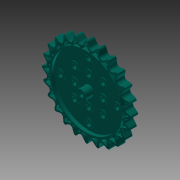
# Autodesk Inventor part: 276-2252
Saved by Autodesk Inventor 2013 (Build 170138000, 138)
## iProperties
Category: Motion
Company: Autodesk Inc.
Created: 2012-03-01
Part Number: 276-2252
Document SubType Name: Modeling
Designer: Autodesk Inc.
Density: 1.42 g/cm^3
Material: Acetal Resin, White
Catalog Web Link: http://www.vexrobotics.com/276-2252.html
Vendor: VEX
Mass: 20.1028 g
Surface Area: 159.433 cm^2
Volume: 14.1569 cm^3
Author: Autodesk Inc.
Autodesk Inventor part; units mm, degrees
ref_plane "YZ Plane" through (0, 0, 0) normal (1, 0, 0) x (0, 1, 0)
ref_plane "XZ Plane" through (0, 0, 0) normal (0, 1, 0) x (-1, 0, 0)
ref_plane "XY Plane" through (0, 0, 0) normal (0, 0, 1) x (1, 0, 0)
sketch "Sketch1" plane through (0, 0, 0) normal (0, 0, 1) x (1, 0, 0)
  circle A0 centre (0, -25.4) radius 2.2225
  circle A1 centre (-12.7, -12.7) radius 2.2225
  circle A2 centre (0, -12.7) radius 2.2225
  circle A3 centre (12.7, -12.7) radius 2.2225
  circle A4 centre (25.4, 0) radius 2.2225
  circle A5 centre (-25.4, 0) radius 2.2225
  circle A6 centre (12.7, 0) radius 2.2225
  circle A7 centre (12.7, 12.7) radius 2.2225
  circle A8 centre (0, 25.4) radius 2.2225
  circle A9 centre (-12.7, 12.7) radius 2.2225
  circle A10 centre (-12.7, 0) radius 2.2225
  circle A11 centre (0, 12.7) radius 2.2225
  line L0 (-1.5875, 1.5875) -> (-1.5875, -1.5875)
  line L1 (-1.5875, -1.5875) -> (1.5875, -1.5875)
  line L2 (1.5875, -1.5875) -> (1.5875, 1.5875)
  line L3 (1.5875, 1.5875) -> (-1.5875, 1.5875)
  arc A12 (35.6037, 6.8783) -> (36.1708, 2.571) centre (37.2166, 4.8997) ccw
  line L4 (36.1708, 2.571) -> (38.9403, 1.3272)
  arc A13 (40.0602, 0.0966) -> (38.9403, 1.3272) centre (38.0859, -0.5752) ccw
  arc A14 (40.0602, -0.0966) -> (40.0602, 0.0966) centre (39.7762, 0) ccw
  arc A15 (38.9403, -1.3272) -> (40.0602, -0.0966) centre (38.0859, 0.5752) ccw
  line L5 (38.9403, -1.3272) -> (36.1708, -2.571)
  arc A16 (36.1708, -2.571) -> (35.6037, -6.8783) centre (37.2166, -4.8997) ccw
  line L6 (35.6037, -6.8783) -> (37.9569, -8.7965)
  arc A17 (38.7202, -10.275) -> (37.9569, -8.7965) centre (36.6392, -10.413) ccw
  arc A18 (38.6701, -10.4617) -> (38.7202, -10.275) centre (38.4208, -10.2948) ccw
  arc A19 (37.2699, -11.3605) -> (38.6701, -10.4617) centre (36.937, -9.3017) ccw
  line L7 (37.2699, -11.3605) -> (34.2729, -11.8451)
  arc A20 (34.2729, -11.8451) -> (32.6103, -15.8588) centre (34.6804, -14.3651) ccw
  line L8 (32.6103, -15.8588) -> (34.3869, -18.3207)
  arc A21 (34.7414, -19.9464) -> (34.3869, -18.3207) centre (32.6957, -19.5411) ccw
  arc A22 (34.6448, -20.1138) -> (34.7414, -19.9464) centre (34.4472, -19.8881) ccw
  arc A23 (33.0597, -20.6195) -> (34.6448, -20.1138) centre (33.2709, -18.5448) ccw
  line L9 (33.0597, -20.6195) -> (30.0393, -20.312)
  arc A24 (30.0393, -20.312) -> (27.3946, -23.7586) centre (29.7807, -22.8515) ccw
  line L10 (27.3946, -23.7586) -> (28.4734, -26.5964)
  arc A25 (28.3952, -28.2585) -> (28.4734, -26.5964) centre (26.524, -27.3375) ccw
  arc A26 (28.2585, -28.3952) -> (28.3952, -28.2585) centre (28.126, -28.126) ccw
  arc A27 (26.5964, -28.4734) -> (28.2585, -28.3952) centre (27.3375, -26.524) ccw
  line L11 (26.5964, -28.4734) -> (23.7586, -27.3946)
  arc A28 (23.7586, -27.3946) -> (20.312, -30.0393) centre (22.8515, -29.7807) ccw
  line L12 (20.312, -30.0393) -> (20.6195, -33.0597)
  arc A29 (20.1138, -34.6448) -> (20.6195, -33.0597) centre (18.5448, -33.2709) ccw
  arc A30 (19.9464, -34.7414) -> (20.1138, -34.6448) centre (19.8881, -34.4472) ccw
  arc A31 (18.3207, -34.3869) -> (19.9464, -34.7414) centre (19.5411, -32.6957) ccw
  line L13 (18.3207, -34.3869) -> (15.8588, -32.6103)
  arc A32 (15.8588, -32.6103) -> (11.8451, -34.2729) centre (14.3651, -34.6804) ccw
  line L14 (11.8451, -34.2729) -> (11.3605, -37.2699)
  arc A33 (10.4617, -38.6701) -> (11.3605, -37.2699) centre (9.3017, -36.937) ccw
  arc A34 (10.275, -38.7202) -> (10.4617, -38.6701) centre (10.2948, -38.4208) ccw
  arc A35 (8.7965, -37.9569) -> (10.275, -38.7202) centre (10.413, -36.6392) ccw
  line L15 (8.7965, -37.9569) -> (6.8783, -35.6037)
  arc A36 (6.8783, -35.6037) -> (2.571, -36.1708) centre (4.8997, -37.2166) ccw
  line L16 (2.571, -36.1708) -> (1.3272, -38.9403)
  arc A37 (0.0966, -40.0602) -> (1.3272, -38.9403) centre (-0.5752, -38.0859) ccw
  arc A38 (-0.0966, -40.0602) -> (0.0966, -40.0602) centre (0, -39.7762) ccw
  arc A39 (-1.3272, -38.9403) -> (-0.0966, -40.0602) centre (0.5752, -38.0859) ccw
  line L17 (-1.3272, -38.9403) -> (-2.571, -36.1708)
  arc A40 (-2.571, -36.1708) -> (-6.8783, -35.6037) centre (-4.8997, -37.2166) ccw
  line L18 (-6.8783, -35.6037) -> (-8.7965, -37.9569)
  arc A41 (-10.275, -38.7202) -> (-8.7965, -37.9569) centre (-10.413, -36.6392) ccw
  arc A42 (-10.4617, -38.6701) -> (-10.275, -38.7202) centre (-10.2948, -38.4208) ccw
  arc A43 (-11.3605, -37.2699) -> (-10.4617, -38.6701) centre (-9.3017, -36.937) ccw
  line L19 (-11.3605, -37.2699) -> (-11.8451, -34.2729)
  arc A44 (-11.8451, -34.2729) -> (-15.8588, -32.6103) centre (-14.3651, -34.6804) ccw
  line L20 (-15.8588, -32.6103) -> (-18.3207, -34.3869)
  arc A45 (-19.9464, -34.7414) -> (-18.3207, -34.3869) centre (-19.5411, -32.6957) ccw
  arc A46 (-20.1138, -34.6448) -> (-19.9464, -34.7414) centre (-19.8881, -34.4472) ccw
  arc A47 (-20.6195, -33.0597) -> (-20.1138, -34.6448) centre (-18.5448, -33.2709) ccw
  line L21 (-20.6195, -33.0597) -> (-20.312, -30.0393)
  arc A48 (-20.312, -30.0393) -> (-23.7586, -27.3946) centre (-22.8515, -29.7807) ccw
  line L22 (-23.7586, -27.3946) -> (-26.5964, -28.4734)
  arc A49 (-28.2585, -28.3952) -> (-26.5964, -28.4734) centre (-27.3375, -26.524) ccw
  arc A50 (-28.3952, -28.2585) -> (-28.2585, -28.3952) centre (-28.126, -28.126) ccw
  arc A51 (-28.4734, -26.5964) -> (-28.3952, -28.2585) centre (-26.524, -27.3375) ccw
  line L23 (-28.4734, -26.5964) -> (-27.3946, -23.7586)
  arc A52 (-27.3946, -23.7586) -> (-30.0393, -20.312) centre (-29.7807, -22.8515) ccw
  line L24 (-30.0393, -20.312) -> (-33.0597, -20.6195)
  arc A53 (-34.6448, -20.1138) -> (-33.0597, -20.6195) centre (-33.2709, -18.5448) ccw
  arc A54 (-34.7414, -19.9464) -> (-34.6448, -20.1138) centre (-34.4472, -19.8881) ccw
  arc A55 (-34.3869, -18.3207) -> (-34.7414, -19.9464) centre (-32.6957, -19.5411) ccw
  line L25 (-34.3869, -18.3207) -> (-32.6103, -15.8588)
  arc A56 (-32.6103, -15.8588) -> (-34.2729, -11.8451) centre (-34.6804, -14.3651) ccw
  line L26 (-34.2729, -11.8451) -> (-37.2699, -11.3605)
  arc A57 (-38.6701, -10.4617) -> (-37.2699, -11.3605) centre (-36.937, -9.3017) ccw
  arc A58 (-38.7202, -10.275) -> (-38.6701, -10.4617) centre (-38.4208, -10.2948) ccw
  arc A59 (-37.9569, -8.7965) -> (-38.7202, -10.275) centre (-36.6392, -10.413) ccw
  line L27 (-37.9569, -8.7965) -> (-35.6037, -6.8783)
  arc A60 (-35.6037, -6.8783) -> (-36.1708, -2.571) centre (-37.2166, -4.8997) ccw
  line L28 (-36.1708, -2.571) -> (-38.9403, -1.3272)
  arc A61 (-40.0602, -0.0966) -> (-38.9403, -1.3272) centre (-38.0859, 0.5752) ccw
  arc A62 (-40.0602, 0.0966) -> (-40.0602, -0.0966) centre (-39.7762, 0) ccw
  arc A63 (-38.9403, 1.3272) -> (-40.0602, 0.0966) centre (-38.0859, -0.5752) ccw
  line L29 (-38.9403, 1.3272) -> (-36.1708, 2.571)
  arc A64 (-36.1708, 2.571) -> (-35.6037, 6.8783) centre (-37.2166, 4.8997) ccw
  line L30 (-35.6037, 6.8783) -> (-37.9569, 8.7965)
  arc A65 (-38.7202, 10.275) -> (-37.9569, 8.7965) centre (-36.6392, 10.413) ccw
  arc A66 (-38.6701, 10.4617) -> (-38.7202, 10.275) centre (-38.4208, 10.2948) ccw
  arc A67 (-37.2699, 11.3605) -> (-38.6701, 10.4617) centre (-36.937, 9.3017) ccw
  line L31 (-37.2699, 11.3605) -> (-34.2729, 11.8451)
  arc A68 (-34.2729, 11.8451) -> (-32.6103, 15.8588) centre (-34.6804, 14.3651) ccw
  line L32 (-32.6103, 15.8588) -> (-34.3869, 18.3207)
  arc A69 (-34.7414, 19.9464) -> (-34.3869, 18.3207) centre (-32.6957, 19.5411) ccw
  arc A70 (-34.6448, 20.1138) -> (-34.7414, 19.9464) centre (-34.4472, 19.8881) ccw
  arc A71 (-33.0597, 20.6195) -> (-34.6448, 20.1138) centre (-33.2709, 18.5448) ccw
  line L33 (-33.0597, 20.6195) -> (-30.0393, 20.312)
  arc A72 (-30.0393, 20.312) -> (-27.3946, 23.7586) centre (-29.7807, 22.8515) ccw
  line L34 (-27.3946, 23.7586) -> (-28.4734, 26.5964)
  arc A73 (-28.3952, 28.2585) -> (-28.4734, 26.5964) centre (-26.524, 27.3375) ccw
  arc A74 (-28.2585, 28.3952) -> (-28.3952, 28.2585) centre (-28.126, 28.126) ccw
  arc A75 (-26.5964, 28.4734) -> (-28.2585, 28.3952) centre (-27.3375, 26.524) ccw
  line L35 (-26.5964, 28.4734) -> (-23.7586, 27.3946)
  arc A76 (-23.7586, 27.3946) -> (-20.312, 30.0393) centre (-22.8515, 29.7807) ccw
  line L36 (-20.312, 30.0393) -> (-20.6195, 33.0597)
  arc A77 (-20.1138, 34.6448) -> (-20.6195, 33.0597) centre (-18.5448, 33.2709) ccw
  arc A78 (-19.9464, 34.7414) -> (-20.1138, 34.6448) centre (-19.8881, 34.4472) ccw
  arc A79 (-18.3207, 34.3869) -> (-19.9464, 34.7414) centre (-19.5411, 32.6957) ccw
  line L37 (-18.3207, 34.3869) -> (-15.8588, 32.6103)
  arc A80 (-15.8588, 32.6103) -> (-11.8451, 34.2729) centre (-14.3651, 34.6804) ccw
  line L38 (-11.8451, 34.2729) -> (-11.3605, 37.2699)
  arc A81 (-10.4617, 38.6701) -> (-11.3605, 37.2699) centre (-9.3017, 36.937) ccw
  arc A82 (-10.275, 38.7202) -> (-10.4617, 38.6701) centre (-10.2948, 38.4208) ccw
  arc A83 (-8.7965, 37.9569) -> (-10.275, 38.7202) centre (-10.413, 36.6392) ccw
  line L39 (-8.7965, 37.9569) -> (-6.8783, 35.6037)
  arc A84 (-6.8783, 35.6037) -> (-2.571, 36.1708) centre (-4.8997, 37.2166) ccw
  line L40 (-2.571, 36.1708) -> (-1.3272, 38.9403)
  arc A85 (-0.0966, 40.0602) -> (-1.3272, 38.9403) centre (0.5752, 38.0859) ccw
  arc A86 (0.0966, 40.0602) -> (-0.0966, 40.0602) centre (0, 39.7762) ccw
  arc A87 (1.3272, 38.9403) -> (0.0966, 40.0602) centre (-0.5752, 38.0859) ccw
  line L41 (1.3272, 38.9403) -> (2.571, 36.1708)
  arc A88 (2.571, 36.1708) -> (6.8783, 35.6037) centre (4.8997, 37.2166) ccw
  line L42 (6.8783, 35.6037) -> (8.7965, 37.9569)
  arc A89 (10.275, 38.7202) -> (8.7965, 37.9569) centre (10.413, 36.6392) ccw
  arc A90 (10.4617, 38.6701) -> (10.275, 38.7202) centre (10.2948, 38.4208) ccw
  arc A91 (11.3605, 37.2699) -> (10.4617, 38.6701) centre (9.3017, 36.937) ccw
  line L43 (11.3605, 37.2699) -> (11.8451, 34.2729)
  arc A92 (11.8451, 34.2729) -> (15.8588, 32.6103) centre (14.3651, 34.6804) ccw
  line L44 (15.8588, 32.6103) -> (18.3207, 34.3869)
  arc A93 (19.9464, 34.7414) -> (18.3207, 34.3869) centre (19.5411, 32.6957) ccw
  arc A94 (20.1138, 34.6448) -> (19.9464, 34.7414) centre (19.8881, 34.4472) ccw
  arc A95 (20.6195, 33.0597) -> (20.1138, 34.6448) centre (18.5448, 33.2709) ccw
  line L45 (20.6195, 33.0597) -> (20.312, 30.0393)
  arc A96 (20.312, 30.0393) -> (23.7586, 27.3946) centre (22.8515, 29.7807) ccw
  line L46 (23.7586, 27.3946) -> (26.5964, 28.4734)
  arc A97 (28.2585, 28.3952) -> (26.5964, 28.4734) centre (27.3375, 26.524) ccw
  arc A98 (28.3952, 28.2585) -> (28.2585, 28.3952) centre (28.126, 28.126) ccw
  arc A99 (28.4734, 26.5964) -> (28.3952, 28.2585) centre (26.524, 27.3375) ccw
  line L47 (28.4734, 26.5964) -> (27.3946, 23.7586)
  arc A100 (27.3946, 23.7586) -> (30.0393, 20.312) centre (29.7807, 22.8515) ccw
  line L48 (30.0393, 20.312) -> (33.0597, 20.6195)
  arc A101 (34.6448, 20.1138) -> (33.0597, 20.6195) centre (33.2709, 18.5448) ccw
  arc A102 (34.7414, 19.9464) -> (34.6448, 20.1138) centre (34.4472, 19.8881) ccw
  arc A103 (34.3869, 18.3207) -> (34.7414, 19.9464) centre (32.6957, 19.5411) ccw
  line L49 (34.3869, 18.3207) -> (32.6103, 15.8588)
  arc A104 (32.6103, 15.8588) -> (34.2729, 11.8451) centre (34.6804, 14.3651) ccw
  line L50 (34.2729, 11.8451) -> (37.2699, 11.3605)
  arc A105 (38.6701, 10.4617) -> (37.2699, 11.3605) centre (36.937, 9.3017) ccw
  arc A106 (38.7202, 10.275) -> (38.6701, 10.4617) centre (38.4208, 10.2948) ccw
  arc A107 (37.9569, 8.7965) -> (38.7202, 10.275) centre (36.6392, 10.413) ccw
  line L51 (37.9569, 8.7965) -> (35.6037, 6.8783)
  point P0 (0, 0)
  point P1 (0, 0)
  constraints: 192 point on circle, 108 centre point, 104 end point
extrude "Extrusion1" add sketch "Sketch1" along normal mid plane 7.62 contours A0 | A1 | A2 | A3 | A4 | A5 | A6 | A7 | A8 | A9 | A10 | A11 | L3 L2 L1 L0 | A12 L4 A13 A14 A15 L5 A16 L6 A17 A18 A19 L7 A20 L8 A21 A22 A23 L9 A24 L10 A25 A26 A27 L11 A28 L12 A29 A30 A31 L13 A32 L14 A33 A34 A35 L15 A36 L16 A37 A38 A39 L17 A40 L18 A41 A42 A43 L19 A44 L20 A45 A46 A47 L21 A48 L22 A49 A50 A51 L23 A52 L24 A53 A54 A55 L25 A56 L26 A57 A58 A59 L27 A60 L28 A61 A62 A63 L29 A64 L30 A65 A66 A67 L31 A68 L32 A69 A70 A71 L33 A72 L34 A73 A74 A75 L35 A76 L36 A77 A78 A79 L37 A80 L38 A81 A82 A83 L39 A84 L40 A85 A86 A87 L41 A88 L42 A89 A90 A91 L43 A92 L44 A93 A94 A95 L45 A96 L46 A97 A98 A99 L47 A100 L48 A101 A102 A103 L49 A104 L50 A105 A106 A107 L51
sketch "Sketch2" plane through (0, 0, 3.81) normal (0, 0, 1) x (1, 0, 0)
  circle A0 centre (0, 0) radius 31.0007
  dimension "d2" = 62.0014
  constraints: 1 centre point, 1 coincident
  measures "d2" diameter of A0
extrude "Extrusion2" cut sketch "Sketch2" against normal blind 2.8194
sketch "Sketch3" plane through (0, 0, 0.9906) normal (0, 0, 1) x (1, 0, 0)
  circle A0 centre (0, 0) radius 31.0007 projected
  circle A1 centre (0, 0) radius 4.4958
  dimension "d5" = 8.9916
  constraints: 1 centre point, 1 coincident
  measures "d5" diameter of A1
extrude "Extrusion3" add sketch "Sketch3" along normal blind 6.9342 contours A1
sketch "Sketch4" plane through (0, 0, 0) normal (1, 0, 0) x (0, 1, 0)
  line L0 (40.0602, -3.81) -> (40.0602, 3.81) projected
  line L1 (36.1708, 3.81) -> (38.9403, 3.81) projected
  line L2 (38.9403, 3.81) -> (40.0602, 3.81) projected
  line L3 (34.2729, 3.81) -> (32.1277, 3.81) projected
  line L4 (36.1708, 3.81) -> (34.6639, 3.81) projected
  line L5 (40.0762, -3.81) -> (40.0762, 3.81) projected
  line L6 (40.0762, 3.81) -> (40.0762, 3.0734)
  line L7 (40.0762, 3.0734) -> (35.8852, 3.81)
  line L8 (35.8852, 3.81) -> (40.0762, 3.81)
  line L9 (0, -5.334) -> (0, 5.334) projected
  point P0 (0, 0)
  point P1 (32.6103, 3.81)
  point P2 (35.6037, 3.81)
  dimension "d8" = 0.7366
  dimension "d9" = 4.191
  constraints: 6 end point, 2 point on line, 1 perpendicular
  measures "d8" distance of L6.end L5.end
  measures "d9" distance of L7.end L5.end
revolve "Revolution1" cut sketch "Sketch4" angle 360 about axis through (0, 0, -10) along (0, 0, 1)
sketch "Sketch5" plane through (0, 0, 3.81) normal (0, 0, 1) x (1, 0, 0)
  line L0 (-36.1588, 0.9321) -> (-35.5563, 1.2027)
  arc A0 (-35.5563, 1.2027) -> (-33.3659, 3.6362) centre (-37.2166, 4.8997) ccw
  line L1 (-33.3659, 3.6362) -> (-32.3113, 3.4974)
  arc A1 (-32.3113, 3.4974) -> (-32.3113, -3.4974) centre (0, 0) ccw
  line L2 (-32.3113, -3.4974) -> (-33.3659, -3.6362)
  arc A2 (-33.3659, -3.6362) -> (-35.5563, -1.2027) centre (-37.2166, -4.8997) ccw
  line L3 (-36.1588, -0.9321) -> (-35.5563, -1.2027)
  line L4 (-38.2342, 0) -> (-36.1588, 0.9321)
  ellipse E0 centre (-37.2141, 4.8919) end of major axis (-34.7934, 5.6895) minor radius 2.5445 (-36.1708, 2.571) -> (-36.0761, 2.6159) ccw
  spline S0 degree 3 poles (-38.9403, 1.3272) (-38.6326, 1.4654) (-38.3249, 1.6036) (-38.0172, 1.7418) (-37.7096, 1.8799) (-37.4018, 2.0181) (-37.0941, 2.1564) (-36.7863, 2.2946) (-36.4786, 2.4328) (-36.1708, 2.571) knots 0 0 0 0 0.333333 0.333333 0.333333 0.666667 0.666667 0.666667 1 1 1 1
  spline S1 degree 3 poles (-40.0602, 0.0966) (-40.0458, 0.1387) (-40.0301, 0.1804) (-39.9033, 0.4873) (-39.7357, 0.7287) (-39.3736, 1.082) (-39.1668, 1.2255) (-38.9403, 1.3272) knots 0 0 0 0 0.076332 0.076332 0.569765 0.569765 1 1 1 1
  spline S2 degree 3 poles (-40.0602, 0.0966) (-40.0709, 0.065) (-40.0762, 0.0316) (-40.0762, -0.0316) (-40.0709, -0.065) (-40.0602, -0.0966) knots 0 0 0 0 0.5 0.5 1 1 1 1
  spline S3 degree 3 poles (-38.9403, -1.3272) (-39.1668, -1.2255) (-39.3736, -1.082) (-39.7357, -0.7287) (-39.9033, -0.4873) (-40.0301, -0.1804) (-40.0458, -0.1387) (-40.0602, -0.0966) knots 0 0 0 0 0.430235 0.430235 0.923668 0.923668 1 1 1 1
  spline S4 degree 3 poles (-38.9403, -1.3272) (-38.6245, -1.469) (-38.3114, -1.6097) (-38.001, -1.7491) (-37.6905, -1.8885) (-37.3828, -2.0267) (-37.0778, -2.1637) (-36.7728, -2.3007) (-36.4704, -2.4365) (-36.1708, -2.571) knots 0 0 0 0 0.333333 0.333333 0.333333 0.666667 0.666667 0.666667 1 1 1 1
  ellipse E1 centre (-37.2137, -4.8911) end of major axis (-34.8027, -5.7161) minor radius 2.5436 (-36.0761, -2.6159) -> (-36.1708, -2.571) ccw
  line L5 (-36.1588, -0.9321) -> (-38.2342, 0)
  constraints: 71 coincident, 12 end point, 6 point on circle, 3 centre point, 1 vertical alignment, 20 other
extrude "Extrusion4" cut sketch "Sketch5" against normal blind 2.8194
fillet "Fillet1" radius 0.3048 12 edges at (-38.2342, 0, 2.1939) (-37.1965, -0.466, 0.9906) (-34.2044, -2.1884, 0.9906) (-34.2044, 2.1884, 0.9906) (-35.8575, 1.0674, 0.9906) (-33.3659, 3.6362, 2.4003) (-32.3113, 3.4974, 2.4003) (-32.3113, -3.4974, 2.4003) (-32.8386, 3.5668, 0.9906) (-32.8386, -3.5668, 0.9906) (-33.3659, -3.6362, 2.4003) (-32.5, 0, 0.9906)
pattern_circular "Circular Pattern1" count 24 over 360 about axis through (0, 0, 0.9906) along (0, 0, 1) of "Extrusion4", "Fillet1"
fillet "Fillet2" radius 0.3048 3 edges at (-31.0007, 0, 0.9906) (-4.4958, 0, 0.9906) (-4.4958, 0, 7.9248)
sketch "Sketch6" plane through (0, 0, 0.9906) normal (0, 0, 1) x (1, 0, 0)
  circle A0 centre (0, 0) radius 30.6959 projected
  circle A1 centre (0, 0) radius 4.8006 projected
  circle A2 centre (-25.4, 0) radius 2.2225 projected
  circle A3 centre (-12.7, -12.7) radius 2.2225 projected
  circle A4 centre (-12.7, 0) radius 2.2225 projected
  circle A5 centre (-12.7, 12.7) radius 2.2225 projected
  circle A6 centre (0, -25.4) radius 2.2225 projected
  circle A7 centre (0, -12.7) radius 2.2225 projected
  circle A8 centre (0, 12.7) radius 2.2225 projected
  circle A9 centre (0, 25.4) radius 2.2225 projected
  circle A10 centre (12.7, 12.7) radius 2.2225 projected
  circle A11 centre (12.7, 0) radius 2.2225 projected
  circle A12 centre (12.7, -12.7) radius 2.2225 projected
  circle A13 centre (25.4, 0) radius 2.2225 projected
  circle A14 centre (-25.4, 0) radius 4.0005
  circle A15 centre (-12.7, -12.7) radius 4.0005
  circle A16 centre (-12.7, 0) radius 4.0005
  circle A17 centre (-12.7, 12.7) radius 4.0005
  circle A18 centre (0, 25.4) radius 4.0005
  circle A19 centre (0, 12.7) radius 4.0005
  circle A20 centre (0, -12.7) radius 4.0005
  circle A21 centre (0, -25.4) radius 4.0005
  circle A22 centre (12.7, -12.7) radius 4.0005
  circle A23 centre (12.7, 0) radius 4.0005
  circle A24 centre (12.7, 12.7) radius 4.0005
  circle A25 centre (25.4, 0) radius 4.0005
  dimension "d25" = 8.001
  constraints: 12 centre point, 12 coincident, 11 equal radius
  measures "d25" diameter of A14
hole "Hole1" at (-12.7, 12.7, 0.9906) at (-25.4, 0, 0.9906) at (-12.7, 0, 0.9906) at (-12.7, -12.7, 0.9906) at (0, -25.4, 0.9906) at (0, -12.7, 0.9906) at (0, 12.7, 0.9906) at (0, 25.4, 0.9906) at (12.7, 12.7, 0.9906) at (12.7, 0, 0.9906) at (12.7, -12.7, 0.9906) at (25.4, 0, 0.9906) direction (0, 0, -1) diameter 4.445 end through all
extrude "Extrusion5" add sketch "Sketch6" along normal blind 0.5842 contours A14 | A15 | A16 | A17 | A18 | A19 | A20 | A21 | A22 | A23 | A24 | A25
mirror "Mirror1" about plane through (0, 0, 0) normal (0, 0, 1) of "Extrusion2", "Extrusion3", "Revolution1", "Extrusion4", "Fillet1", "Circular Pattern1", "Fillet2", "Extrusion5"
extrude "Extrusion6" cut sketch "Sketch1" against normal up to surface (15.8496 mm away) from surface at 7.9248 contours L3 L2 L1 L0
sketch "Sketch7" plane through (0, 0, 7.9248) normal (0, 0, 1) x (1, 0, 0)
  circle A0 centre (0, 0) radius 4.191 projected
  circle A1 centre (0, 0) radius 1.5875
  constraints: 1 centre point, 1 coincident
surface extrude "ExtrusionSrf1" sketch "Sketch7" against normal up to surface (15.8496 mm away) shown no curves A1
body "Solid1"
body "Srf1"
